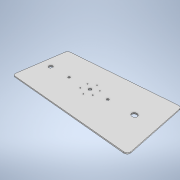
# Autodesk Inventor part: antenna-mount
Saved by Autodesk Inventor 2020.2 (Build 242310000, 310)
## iProperties
Created: 2019-07-22
Part Number: antenna-mount
Material: Generic
Document SubType Name: Modeling
Designer: Nicholas
Density: 1 g/cm^3
Appearance: Default
Author: Nicholas
Autodesk Inventor part; units mm, degrees
ref_plane "YZ Plane" through (0, 0, 0) normal (1, 0, 0) x (0, 1, 0)
ref_plane "XZ Plane" through (0, 0, 0) normal (0, 1, 0) x (-1, 0, 0)
ref_plane "Work Plane4" through (60.2613, -49.3334, 0) normal (0, 1, 0) x (1, 0, 0)
sketch "dimensions" plane through (60.2613, -49.3334, 0) normal (0, 1, 0) x (1, 0, 0)
  line L0 (-254, 127) -> (254, 127)
  line L1 (254, 127) -> (254, -127)
  line L2 (254, -127) -> (-254, -127)
  line L3 (-254, -127) -> (-254, 127)
  line L4 (-254, 127) -> (254, -127) construction
  line L5 (254, 127) -> (-254, -127) construction
  line L6 (-254, 0) -> (254, 0) construction
  circle A0 centre (177.8, 0) radius 10.5
  circle A1 centre (177.8, 0) radius 47.15 construction
  circle A2 centre (-203.2, 0) radius 9.5
  circle A3 centre (-203.2, 0) radius 23.9 construction
  circle A4 centre (2.7586, -32.2833) radius 2.1
  circle A5 centre (28.0468, -16.173) radius 2.1
  circle A6 centre (28.0468, 16.2948) radius 2.1
  circle A7 centre (-0.0711, 32.5287) radius 2.1
  circle A8 centre (-28.1891, 16.2948) radius 2.1
  circle A9 centre (-28.1891, -16.173) radius 2.1
  circle A10 centre (-0.0711, 0.0609) radius 6.35
  line L7 (177.8, 0) -> (-203.2, 0) construction
  circle A11 centre (76.2, 0) radius 5
  circle A12 centre (-101.6, 0) radius 5
  dimension "d1" = 508
  dimension "d2" = 254
  dimension "d3" = 21
  dimension "d4" = 94.3
  dimension "d6" = 19
  dimension "d7" = 47.8
  dimension "d32" = 10
  dimension "d34" = 101.6
  dimension "d35" = 10
  dimension "d36" = 101.6
  constraints: 16 end point, 13 centre point, 4 point on line, 2 coincident, 2 midpoint, 2 parallel, 1 collinear, 1 horizontal, 1 perpendicular
  measures "d1" distance of L1.end L2.end
  measures "d2" distance of L0.end L1.end
  measures "d3" diameter of A0
  measures "d4" diameter of A1
  measures "d6" diameter of A2
  measures "d7" diameter of A3
  measures "d32" diameter of A11
  measures "d34" distance of A11.centre A0.centre
  measures "d35" diameter of A12
  measures "d36" distance of A12.centre A2.centre
extrude "Extrusion5" add sketch "dimensions" along normal blind 5 contours L0 L1 L2 L3 | A11 | A12
fillet "Fillet6" radius 12.7 4 edges at (314.2613, -46.8334, -127) (-193.7387, -46.8334, -127) (-193.7387, -46.8334, 127) (314.2613, -46.8334, 127)
extrude "Extrusion6" cut sketch "dimensions" along normal up to next contours A11 | A12
equation "\"d37\" = d36"
body "Solid4"
